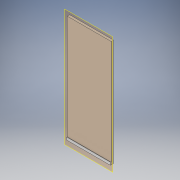
# Autodesk Inventor part: wall
Saved by Autodesk Inventor 2018 (Build 220112000, 112)
## iProperties
Created: 2018-11-24
Part Number: wall
Material: Generic
Document SubType Name: Modeling
Designer: Gage
Density: 1 g/cm^3
Appearance: Default
Author: Gage
Autodesk Inventor part; units mm, degrees
ref_plane "YZ Plane" through (0, 0, 0) normal (1, 0, 0) x (0, 1, 0)
ref_plane "XZ Plane" through (0, 0, 0) normal (0, 1, 0) x (-1, 0, 0)
ref_plane "XY Plane" through (0, 0, 0) normal (0, 0, 1) x (1, 0, 0)
sketch "Sketch1" plane through (0, 0, 0) normal (0, 0, 1) x (1, 0, 0)
  line L0 (-12.7, 30.861) -> (12.7, 30.861)
  line L1 (12.7, 30.861) -> (12.7, -30.861)
  line L2 (12.7, -30.861) -> (-12.7, -30.861)
  line L3 (-12.7, -30.861) -> (-12.7, 30.861)
  line L4 (-12.7, 30.861) -> (12.7, -30.861) construction
  line L5 (12.7, 30.861) -> (-12.7, -30.861) construction
  point P0 (0, 0)
  dimension "d0" = 25.4
  dimension "d1" = 61.722
  constraints: 12 end point, 2 midpoint, 2 parallel, 1 horizontal, 1 perpendicular
  measures "d0" distance of L1.end L2.end
  measures "d1" distance of L0.end L1.end
extrude "Extrusion1" add sketch "Sketch1" along normal blind 1.397
sketch "Sketch3" plane through (12.7, -30.861, 0) normal (1, 0, 0) x (0, 0, -1)
  line L0 (0, 61.722) -> (0, 0) projected
  line L1 (0, 61.722) -> (-1.397, 61.722) projected
  line L2 (-1.397, 0) -> (-1.397, 61.722) projected
  line L3 (0, 0) -> (-1.397, 0) projected
  line L4 (-1.397, 0) -> (-1.905, 0)
  line L5 (-1.397, 0) -> (-1.397, 1.27)
  line L6 (-1.397, 53.34) -> (-1.397, 0) projected
  line L7 (-1.651, 1.27) -> (-1.397, 1.27)
  line L8 (-1.651, 1.27) -> (-1.905, 0)
  point P0 (0, 30.861)
  dimension "d8" = 0.508
  dimension "d9" = 1.27
  dimension "d10" = 0.254
  constraints: 8 end point, 2 horizontal, 1 collinear
  measures "d8" distance of L2.start L4.end
  measures "d9" distance of L2.start L5.end
  measures "d10" distance of L7.start L5.end
ref_plane "Work Plane1" through (0, 0, 1.651) normal (0, 0, 1) x (1, 0, 0)
sketch "Sketch6" plane through (0, 0, 1.651) normal (0, 0, 1) x (1, 0, 0)
  line L0 (12.7, -29.591) -> (12.7, -30.861) projected
  line L1 (12.7, -30.861) -> (12.7, 30.861) projected
  line L2 (12.7, -30.226) -> (-12.7, -30.226)
  line L3 (-12.7, -30.861) -> (12.7, -30.861) projected
  line L4 (-12.7, -30.861) -> (12.7, -30.861) projected
  point P0 (0, 0)
  dimension "d12" = 0.635
  constraints: 2 end point, 1 horizontal, 1 point on line
  measures "d12" distance between parallel lines of L3 L2
sweep "Sweep1" add profiles "Sketch3" path "Sketch6" path curves L2 contours L4 L8 L7 L2
body "Solid1"
